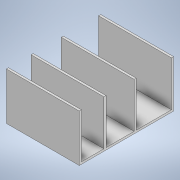
# Autodesk Inventor part: Part1
Saved by Autodesk Inventor 2022.2 (Build 262287000, 287)
## iProperties
Created: 2022-02-28
Part Number: Part1
Material: Generic
Document SubType Name: Modeling
Designer: PRASHANTH
Density: 1 g/cm^3
Appearance: Default
Author: PRASHANTH
Autodesk Inventor part; units mm, degrees
ref_plane "YZ Plane" through (0, 0, 0) normal (1, 0, 0) x (0, 1, 0)
ref_plane "XZ Plane" through (0, 0, 0) normal (0, 1, 0) x (-1, 0, 0)
ref_plane "XY Plane" through (0, 0, 0) normal (0, 0, 1) x (1, 0, 0)
sketch "Sketch1" plane through (0, 0, 0) normal (1, 0, 0) x (0, 1, 0)
  line L0 (-57.5, 47.1421) -> (52.5, 47.1421)
  line L1 (52.5, -172.8579) -> (-57.5, -172.8579)
  line L2 (-57.5, -172.8579) -> (-57.5, 47.1421)
  line L3 (52.5, 42.1421) -> (-52.5, 42.1421)
  line L4 (-52.5, -167.8579) -> (52.5, -167.8579)
  line L5 (52.5, -10.3579) -> (-52.5, -10.3579)
  line L6 (-52.5, -15.3579) -> (52.5, -15.3579)
  line L7 (52.5, -80.8579) -> (-52.5, -80.8579)
  line L8 (-52.5, -85.8579) -> (52.5, -85.8579)
  line L9 (-52.5, 42.1421) -> (-52.5, -10.3579)
  line L10 (-52.5, -15.3579) -> (-52.5, -80.8579)
  line L11 (-52.5, -85.8579) -> (-52.5, -167.8579)
  line L12 (52.5, 47.1421) -> (52.5, 42.1421)
  line L13 (52.5, -10.3579) -> (52.5, -15.3579)
  line L14 (52.5, -80.8579) -> (52.5, -85.8579)
  line L15 (52.5, -167.8579) -> (52.5, -172.8579)
  point P0 (0, 0)
  point P1 (0, -85.8579)
  dimension "d4" = 52.5
  dimension "d5" = 5
  dimension "d6" = 65.5
  dimension "d7" = 5
  dimension "d10" = 82
  constraints: 32 end point, 7 perpendicular, 4 equal length, 1 horizontal, 1 midpoint, 1 point on line
  measures "d4" distance between parallel lines of L5 L3
  measures "d5" distance between parallel lines of L6 L5
  measures "d6" distance between parallel lines of L7 L6
  measures "d7" distance from line of point (0, -85.858) L7
  measures "d10" distance between parallel lines of L4 L8
extrude "Extrusion1" add sketch "Sketch1" along normal blind 170
sketch "Sketch2" plane through (0, -52.5, 42.1421) normal (0, 1, 0) x (1, 0, 0)
  line L0 (0, 210) -> (170, 210) projected
  circle A0 centre (85, 169.7321) radius 7.5
  circle A1 centre (85, 91.3679) radius 7.5
  circle A2 centre (85, 28.7449) radius 7.5
  point P0 (0, 42.1421)
  constraints: 3 centre point
extrude "Extrusion2" cut sketch "Sketch2" against normal blind 5
body "Solid1"
